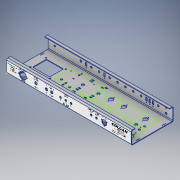
# Autodesk Inventor part: mainChassis
Saved by Autodesk Inventor 2018.3 (Build 223284000, 284)
## iProperties
Created: 2019-02-19
Part Number: mainChassis
Material: Aluminum 6061
Document SubType Name: Sheet Metal
Designer: RCCol
Density: 2.7 g/cm^3
Sheet Metal Rule: .125 thick aluminum
Appearance: Aluminum - Flat
Flat Pattern Width: 34.7497 cm
Flat Pattern Length: 60.325 cm
Flat Pattern Area: 2096.27 cm^2
Sheet Metal Width: 13.681 in
Sheet Metal Length: 23.750 in
Sheet Metal Area: 324.923 in^2
Author: RCCol
Autodesk Inventor part; units mm, degrees
(part 1 of 3)
ref_plane "YZ Plane" through (0, 0, 0) normal (1, 0, 0) x (0, 1, 0)
ref_plane "XZ Plane" through (0, 0, 0) normal (0, 1, 0) x (-1, 0, 0)
ref_plane "XY Plane" through (0, 0, 0) normal (0, 0, 1) x (1, 0, 0)
sketch "Sketch1" plane through (0, 0, 0) normal (0, 1, 0) x (-1, 0, 0)
  line L0 (0, 0) -> (-603.25, 0)
  line L1 (-603.25, 0) -> (-603.25, -204.47)
  line L2 (-603.25, -204.47) -> (0, -204.47)
  line L3 (0, -204.47) -> (0, 0)
  line L4 (0, 0) -> (-254, 0)
  line L5 (0, -79.375) -> (0, 0)
  dimension "d0" = 603.25
  dimension "d1" = 204.47
  constraints: 12 end point, 2 horizontal, 2 parallel, 1 perpendicular
  measures "d0" distance of L2.end L1.end
  measures "d1" distance of L1.end L0.end
extrude "Plate1" add sketch "Sketch1" along normal blind 3.175
sketch "Sketch2" plane through (0, 3.175, 0) normal (0, 1, 0) x (1, 0, 0)
  line L0 (41.3, 154.94) -> (117.45, 154.94)
  arc A0 (120.65, 151.74) -> (117.45, 154.94) centre (117.45, 151.74) ccw
  line L1 (41.3, 87.63) -> (117.45, 87.63)
  arc A1 (117.45, 87.63) -> (120.65, 90.83) centre (117.45, 90.83) ccw
  line L2 (38.1, 151.74) -> (38.1, 90.83)
  arc A2 (41.3, 154.94) -> (38.1, 151.74) centre (41.3, 151.74) ccw
  arc A3 (38.1, 90.83) -> (41.3, 87.63) centre (41.3, 90.83) ccw
  circle A4 centre (31.75, 177.5295) radius 1.5
  line L3 (120.65, 151.74) -> (120.65, 90.83)
  circle A5 centre (147.375, 75.2475) radius 1.65
  circle A6 centre (147.375, 164.1475) radius 1.65
  circle A7 centre (185.1575, 138.7475) radius 2.65
  circle A8 centre (185.1575, 178.435) radius 2.65
  circle A9 centre (235.9575, 87.1648) radius 2.65
  circle A10 centre (243.895, 87.1648) radius 2.65
  circle A11 centre (235.9575, 169.7148) radius 2.65
  circle A12 centre (243.895, 169.7148) radius 2.65
  circle A13 centre (259.135, 75.2475) radius 1.65
  circle A14 centre (259.135, 164.1475) radius 1.65
  circle A15 centre (551.549, 97.0569) radius 1.65
  arc A16 (187.6575, 169.4256) -> (182.6575, 169.4256) centre (185.1575, 169.4256) ccw
  arc A17 (182.6575, 164.4256) -> (187.6575, 164.4256) centre (185.1575, 164.4256) ccw
  line L4 (187.6575, 169.4256) -> (187.6575, 164.4256)
  line L5 (182.6575, 169.4256) -> (182.6575, 164.4256)
  arc A18 (187.6575, 90.4475) -> (182.6575, 90.4475) centre (185.1575, 90.4475) ccw
  arc A19 (182.6575, 85.4475) -> (187.6575, 85.4475) centre (185.1575, 85.4475) ccw
  line L6 (187.6575, 90.4475) -> (187.6575, 85.4475)
  line L7 (182.6575, 90.4475) -> (182.6575, 85.4475)
  arc A20 (308.1355, 175.935) -> (308.1355, 180.935) centre (308.1355, 178.435) ccw
  arc A21 (301.1355, 180.935) -> (301.1355, 175.935) centre (301.1355, 178.435) ccw
  line L8 (308.1355, 175.935) -> (301.1355, 175.935)
  line L9 (308.1355, 180.935) -> (301.1355, 180.935)
  arc A22 (243.048, 175.935) -> (243.048, 180.935) centre (243.048, 178.435) ccw
  arc A23 (236.048, 180.935) -> (236.048, 175.935) centre (236.048, 178.435) ccw
  line L10 (243.048, 175.935) -> (236.048, 175.935)
  line L11 (243.048, 180.935) -> (236.048, 180.935)
  arc A24 (298.195, 167.2148) -> (298.195, 172.2148) centre (298.195, 169.7148) ccw
  arc A25 (291.195, 172.2148) -> (291.195, 167.2148) centre (291.195, 169.7148) ccw
  line L12 (298.195, 167.2148) -> (291.195, 167.2148)
  line L13 (298.195, 172.2148) -> (291.195, 172.2148)
  arc A26 (308.1355, 110.435) -> (308.1355, 115.435) centre (308.1355, 112.935) ccw
  arc A27 (301.1355, 115.435) -> (301.1355, 110.435) centre (301.1355, 112.935) ccw
  line L14 (308.1355, 110.435) -> (301.1355, 110.435)
  line L15 (308.1355, 115.435) -> (301.1355, 115.435)
  arc A28 (308.1355, 99.735) -> (308.1355, 104.735) centre (308.1355, 102.235) ccw
  arc A29 (301.1355, 104.735) -> (301.1355, 99.735) centre (301.1355, 102.235) ccw
  line L16 (308.1355, 99.735) -> (301.1355, 99.735)
  line L17 (308.1355, 104.735) -> (301.1355, 104.735)
  arc A30 (243.048, 110.435) -> (243.048, 115.435) centre (243.048, 112.935) ccw
  arc A31 (236.048, 115.435) -> (236.048, 110.435) centre (236.048, 112.935) ccw
  line L18 (243.048, 110.435) -> (236.048, 110.435)
  line L19 (243.048, 115.435) -> (236.048, 115.435)
  arc A32 (243.048, 99.735) -> (243.048, 104.735) centre (243.048, 102.235) ccw
  arc A33 (236.048, 104.735) -> (236.048, 99.735) centre (236.048, 102.235) ccw
  line L20 (243.048, 99.735) -> (236.048, 99.735)
  line L21 (243.048, 104.735) -> (236.048, 104.735)
  arc A34 (298.195, 84.6648) -> (298.195, 89.6648) centre (298.195, 87.1648) ccw
  arc A35 (291.195, 89.6648) -> (291.195, 84.6648) centre (291.195, 87.1648) ccw
  line L22 (298.195, 84.6648) -> (291.195, 84.6648)
  line L23 (298.195, 89.6648) -> (291.195, 89.6648)
  circle A36 centre (237.6, 35.56) radius 15.1
  arc A37 (239.251, 57.4158) -> (238.6557, 58.0111) centre (238.6557, 57.4158) ccw
  arc A38 (238.6557, 53.1089) -> (239.251, 53.7042) centre (238.6557, 53.7042) ccw
  line L24 (239.251, 53.7042) -> (239.251, 57.4158)
  arc A39 (236.5443, 58.0111) -> (235.949, 57.4158) centre (236.5443, 57.4158) ccw
  line L25 (235.949, 53.7042) -> (235.949, 57.4158)
  line L26 (238.6557, 58.0111) -> (236.5443, 58.0111)
  line L27 (238.6557, 53.1089) -> (236.5443, 53.1089)
  arc A40 (235.949, 53.7042) -> (236.5443, 53.1089) centre (236.5443, 53.7042) ccw
  arc A41 (239.251, 17.4158) -> (238.6557, 18.0111) centre (238.6557, 17.4158) ccw
  arc A42 (238.6557, 13.1089) -> (239.251, 13.7042) centre (238.6557, 13.7042) ccw
  line L28 (239.251, 13.7042) -> (239.251, 17.4158)
  arc A43 (236.5443, 18.0111) -> (235.949, 17.4158) centre (236.5443, 17.4158) ccw
  line L29 (235.949, 13.7042) -> (235.949, 17.4158)
  line L30 (238.6557, 18.0111) -> (236.5443, 18.0111)
  line L31 (238.6557, 13.1089) -> (236.5443, 13.1089)
  arc A44 (235.949, 13.7042) -> (236.5443, 13.1089) centre (236.5443, 13.7042) ccw
  circle A45 centre (174.1, 35.56) radius 15.1
  arc A46 (175.751, 57.4158) -> (175.1557, 58.0111) centre (175.1557, 57.4158) ccw
  arc A47 (175.1557, 53.1089) -> (175.751, 53.7042) centre (175.1557, 53.7042) ccw
  line L32 (175.751, 53.7042) -> (175.751, 57.4158)
  arc A48 (173.0443, 58.0111) -> (172.449, 57.4158) centre (173.0443, 57.4158) ccw
  line L33 (172.449, 53.7042) -> (172.449, 57.4158)
  line L34 (175.1557, 58.0111) -> (173.0443, 58.0111)
  line L35 (175.1557, 53.1089) -> (173.0443, 53.1089)
  arc A49 (172.449, 53.7042) -> (173.0443, 53.1089) centre (173.0443, 53.7042) ccw
  arc A50 (175.751, 17.4158) -> (175.1557, 18.0111) centre (175.1557, 17.4158) ccw
  arc A51 (175.1557, 13.1089) -> (175.751, 13.7042) centre (175.1557, 13.7042) ccw
  line L36 (175.751, 13.7042) -> (175.751, 17.4158)
  arc A52 (173.0443, 18.0111) -> (172.449, 17.4158) centre (173.0443, 17.4158) ccw
  line L37 (172.449, 13.7042) -> (172.449, 17.4158)
  line L38 (175.1557, 18.0111) -> (173.0443, 18.0111)
  line L39 (175.1557, 13.1089) -> (173.0443, 13.1089)
  arc A53 (172.449, 13.7042) -> (173.0443, 13.1089) centre (173.0443, 13.7042) ccw
  circle A54 centre (110.6, 35.56) radius 15.1
  arc A55 (112.251, 57.4158) -> (111.6557, 58.0111) centre (111.6557, 57.4158) ccw
  arc A56 (111.6557, 53.1089) -> (112.251, 53.7042) centre (111.6557, 53.7042) ccw
  line L40 (112.251, 53.7042) -> (112.251, 57.4158)
  arc A57 (109.5443, 58.0111) -> (108.949, 57.4158) centre (109.5443, 57.4158) ccw
  line L41 (108.949, 53.7042) -> (108.949, 57.4158)
  line L42 (111.6557, 58.0111) -> (109.5443, 58.0111)
  line L43 (111.6557, 53.1089) -> (109.5443, 53.1089)
  arc A58 (108.949, 53.7042) -> (109.5443, 53.1089) centre (109.5443, 53.7042) ccw
  arc A59 (112.251, 17.4158) -> (111.6557, 18.0111) centre (111.6557, 17.4158) ccw
  arc A60 (111.6557, 13.1089) -> (112.251, 13.7042) centre (111.6557, 13.7042) ccw
  line L44 (112.251, 13.7042) -> (112.251, 17.4158)
  arc A61 (109.5443, 18.0111) -> (108.949, 17.4158) centre (109.5443, 17.4158) ccw
  line L45 (108.949, 13.7042) -> (108.949, 17.4158)
  line L46 (111.6557, 18.0111) -> (109.5443, 18.0111)
  line L47 (111.6557, 13.1089) -> (109.5443, 13.1089)
  arc A62 (108.949, 13.7042) -> (109.5443, 13.1089) centre (109.5443, 13.7042) ccw
  circle A63 centre (47.1, 35.56) radius 15.1
  arc A64 (48.751, 57.4158) -> (48.1557, 58.0111) centre (48.1557, 57.4158) ccw
  arc A65 (48.1557, 53.1089) -> (48.751, 53.7042) centre (48.1557, 53.7042) ccw
  line L48 (48.751, 53.7042) -> (48.751, 57.4158)
  arc A66 (46.0443, 58.0111) -> (45.449, 57.4158) centre (46.0443, 57.4158) ccw
  line L49 (45.449, 53.7042) -> (45.449, 57.4158)
  line L50 (48.1557, 58.0111) -> (46.0443, 58.0111)
  line L51 (48.1557, 53.1089) -> (46.0443, 53.1089)
  arc A67 (45.449, 53.7042) -> (46.0443, 53.1089) centre (46.0443, 53.7042) ccw
  arc A68 (48.751, 17.4158) -> (48.1557, 18.0111) centre (48.1557, 17.4158) ccw
  arc A69 (48.1557, 13.1089) -> (48.751, 13.7042) centre (48.1557, 13.7042) ccw
  line L52 (48.751, 13.7042) -> (48.751, 17.4158)
  arc A70 (46.0443, 18.0111) -> (45.449, 17.4158) centre (46.0443, 17.4158) ccw
  line L53 (45.449, 13.7042) -> (45.449, 17.4158)
  line L54 (48.1557, 18.0111) -> (46.0443, 18.0111)
  line L55 (48.1557, 13.1089) -> (46.0443, 13.1089)
  arc A71 (45.449, 13.7042) -> (46.0443, 13.1089) centre (46.0443, 13.7042) ccw
  circle A72 centre (159.7575, 106.3403) radius 4.8
  circle A73 centre (212.2, 93.5148) radius 4.8
  circle A74 centre (309.5568, 135.335) radius 6.35
  circle A75 centre (234.6268, 135.335) radius 6.35
  circle A76 centre (269.35, 26.9408) radius 1.651
  circle A77 centre (515.9375, 36.5125) radius 9.525
  circle A78 centre (515.3168, 50.7865) radius 1.651
  circle A79 centre (516.5582, 22.2385) radius 1.651
  circle A80 centre (530.225, 142.875) radius 9.525
  circle A81 centre (530.225, 157.1625) radius 1.651
  circle A82 centre (530.225, 128.5875) radius 1.651
  circle A83 centre (425.45, 142.875) radius 9.525
  circle A84 centre (425.45, 157.1625) radius 1.651
  circle A85 centre (425.45, 128.5875) radius 1.651
  circle A86 centre (363.5375, 142.875) radius 9.525
  circle A87 centre (363.5375, 157.1625) radius 1.651
  circle A88 centre (363.5375, 128.5875) radius 1.651
  circle A89 centre (336.55, 37.1475) radius 9.525
  circle A90 centre (336.757, 22.8615) radius 1.651
  circle A91 centre (336.343, 51.4335) radius 1.651
  circle A92 centre (205.85, 26.9408) radius 1.651
  circle A93 centre (78.85, 26.9408) radius 1.651
  circle A94 centre (78.85, 63.0879) radius 1.651
  circle A95 centre (19.05, 63.0879) radius 1.651
  circle A96 centre (142.35, 26.035) radius 1.651
  circle A97 centre (22.225, 20.5908) radius 1.651
  arc A98 (187.6575, 104.4569) -> (182.6575, 104.4569) centre (185.1575, 104.4569) ccw
  arc A99 (182.6575, 99.4569) -> (187.6575, 99.4569) centre (185.1575, 99.4569) ccw
  line L56 (187.6575, 104.4569) -> (187.6575, 99.4569)
  line L57 (182.6575, 104.4569) -> (182.6575, 99.4569)
  circle A100 centre (193.85, 60.5908) radius 1.65
  circle A101 centre (217.85, 60.5908) radius 1.65
  circle A102 centre (205.85, 60.5908) radius 4.826
  circle A103 centre (137.16, 62.3578) radius 1.651
  circle A104 centre (558.8, 109.5375) radius 4.826
  circle A105 centre (558.8, 84.1375) radius 4.826
  circle A106 centre (518.6157, 61.2782) radius 2.3813
  circle A107 centre (529.5939, 97.3765) radius 6.35
  circle A108 centre (563.0654, 61.4489) radius 2.3813
  circle A109 centre (31.75, 159.385) radius 3.175
  circle A110 centre (127, 159.385) radius 3.175
  circle A111 centre (31.75, 83.185) radius 3.175
  circle A112 centre (127, 83.185) radius 3.175
  circle A113 centre (565.8874, 37.1475) radius 9.525
  circle A114 centre (565.8026, 51.4347) radius 1.651
  circle A115 centre (565.9721, 22.8603) radius 1.651
  circle A116 centre (78.85, 35.56) radius 3.2385
  circle A117 centre (142.35, 35.56) radius 3.2385
  circle A118 centre (205.85, 35.56) radius 3.2385
  circle A119 centre (269.35, 35.56) radius 3.2385
  circle A120 centre (6.35, 165.735) radius 2.667
  circle A121 centre (6.35, 158.3944) radius 1.5875
  circle A122 centre (6.35, 173.0756) radius 1.5875
  circle A123 centre (6.35, 38.735) radius 2.667
  circle A124 centre (6.35, 31.3944) radius 1.5875
  circle A125 centre (6.35, 46.0756) radius 1.5875
  circle A126 centre (596.9, 38.735) radius 2.667
  circle A127 centre (596.9, 46.0756) radius 1.5875
  circle A128 centre (596.9, 31.3944) radius 1.5875
  circle A129 centre (596.9, 165.735) radius 2.667
  circle A130 centre (596.9, 173.0756) radius 1.5875
  circle A131 centre (596.9, 158.3944) radius 1.5875
  circle A132 centre (257.175, 61.9125) radius 3.2385
  circle A133 centre (117.45, 90.83) radius 3.2
  circle A134 centre (41.3, 90.83) radius 3.2
  circle A135 centre (41.3, 151.74) radius 3.2
  circle A136 centre (117.45, 151.74) radius 3.2
  line L58 (117.45, 87.63) -> (41.3, 87.63)
  line L59 (41.3, 87.63) -> (41.3, 154.94)
  line L60 (41.3, 154.94) -> (117.45, 154.94)
  line L61 (117.45, 154.94) -> (117.45, 87.63)
  line L62 (38.1, 90.83) -> (120.65, 90.83)
  line L63 (120.65, 90.83) -> (120.65, 151.74)
  line L64 (120.65, 151.74) -> (38.1, 151.74)
  line L65 (38.1, 151.74) -> (38.1, 90.83)
  line L66 (481.5672, 92.8982) -> (586.4692, 92.8982) construction
  line L67 (586.4692, 92.8982) -> (586.4692, 13.4373) construction
  line L68 (586.4692, 13.4373) -> (481.5672, 13.4373) construction
  line L69 (481.5672, 13.4373) -> (481.5672, 92.8982) construction
  line L70 (327.7837, 182.0084) -> (581.4999, 182.0084) construction
  line L71 (581.4999, 182.0084) -> (581.4999, 102.7644) construction
  line L72 (581.4999, 102.7644) -> (327.7837, 102.7644) construction
  line L73 (327.7837, 102.7644) -> (327.7837, 182.0084) construction
  line L74 (264.3245, 93.0716) -> (416.75, 93.5014) construction
  line L75 (416.75, 93.5014) -> (416.9742, 13.9788) construction
  line L76 (416.9742, 13.9788) -> (264.5487, 13.549) construction
  line L77 (264.5487, 13.549) -> (264.3245, 93.0716) construction
  circle A137 centre (298.195, 37.1475) radius 9.525
  circle A138 centre (298.3621, 51.434) radius 1.651
  circle A139 centre (298.0279, 22.861) radius 1.651
  line L78 (137.2091, 179.1073) -> (295.4903, 179.1073) construction
  line L79 (295.4903, 179.1073) -> (295.4903, 100.0089) construction
  line L80 (295.4903, 100.0089) -> (137.2091, 100.0089) construction
  line L81 (137.2091, 100.0089) -> (137.2091, 179.1073) construction
  circle A140 centre (436.5625, 46.0375) radius 14.9987
  circle A141 centre (436.5625, 68.8975) radius 1.651
  circle A142 centre (436.5625, 23.1775) radius 1.651
  dimension "GapSize" = 3.175
  dimension "d353" = 29.9974
  dimension "d378" = 3.302
  dimension "d379" = 3.302
  dimension "d417" = 22.86
  dimension "d418" = 22.86
  constraints: 141 centre point, 132 end point, 116 point on circle, 4 coincident, 4 parallel, 2 horizontal, 2 horizontal alignment, 2 perpendicular, 2 point on line, 12 other
  measures "d353" diameter of A140
  measures "d378" diameter of A141
  measures "d379" diameter of A142
  measures "d417" distance of A141.centre A140.centre
  measures "d418" distance of A140.centre A142.centre
extrude "Cut1" cut sketch "Sketch2" against normal blind 3.175 contours L59 L64 A2 | L0 A136 L64 A135 | A135 L64 L59 | L61 L64 A136 | A0 L64 L61 | A135 L59 A134 L2 | L64 L59 A135 | L64 A136 L61 A133 L62 A134 L59 A135 | A135 L59 L64 | L3 A133 L61 A136 | A136 L61 L64 | L64 L61 A136 | L62 L59 A3 | A134 L59 L62 | L62 L61 A133 | A1 L61 L62 | A134 L62 A133 L1 | L59 L62 A134 | A134 L62 L59 | A133 L62 L61 | L61 L62 A133 | A5 | A6 | A7 | A8 | A9 | A10 | A11 | A12 | A13 | A14 | A15 | L4 A17 L5 A16 | L6 A19 L7 A18 | L8 A21 L9 A20 | L10 A23 L11 A22 | L12 A25 L13 A24 | L14 A27 L15 A26 | L16 A29 L17 A28 | L18 A31 L19 A30 | L20 A33 L21 A32 | L22 A35 L23 A34 | A36 | L24 A38 L27 A40 L25 A39 L26 A37 | L28 A42 L31 A44 L29 A43 L30 A41 | A45 | L32 A47 L35 A49 L33 A48 L34 A46 | L36 A51 L39 A53 L37 A52 L38 A50 | A54 | L40 A56 L43 A58 L41 A57 L42 A55 | L44 A60 L47 A62 L45 A61 L46 A59 | A63 | L48 A65 L51 A67 L49 A66 L50 A64 | L52 A69 L55 A71 L53 A70 L54 A68 | A72 | A73 | A74 | A75 | A76 | A77 | A78 | A79 | A80 | A81 | A82 | A83 | A84 | A85 | A86 | A87 | A88 | A89 | A90 | A91 | A92 | A93 | A94 | A95 | A96 | A97 | L56 A99 L57 A98 | A100 | A101 | A102 | A103 | A104 | A105 | A106 | A107 | A108 | A109 | A110 | A111 | A112 | A113 | A114 | A115 | A116 | A117 | A118 | A119 | A120 | A121 | A122 | A123 | A124 | A125 | A126 | A127 | A128 | A129 | A130 | A131 | A132 | A137 | A138 | A139 | A140 | A141 | A142
sketch "Sketch3" plane through (603.25, 0, -3.175) normal (0, 0, 1) x (1, 0, 0)
  line L0 (-603.25, 0) -> (0, 0)
  line L1 (0, 0) -> (0, 63.5)
  line L2 (0, 63.5) -> (-603.25, 63.5)
  line L3 (-603.25, 63.5) -> (-603.25, 0)
  constraints: 6 end point, 1 horizontal, 1 perpendicular, 1 vertical
edge flange "Flange1" height 63.5 angle 90 thickness 3.175 bend radius 3.175 thickness toward (0, 0, 1) relief straight relief width 3.175 relief depth 1.5875 edges at (301.625, 3.175, 0) wall of the first edge with corners at (0, 0, -3.175) (603.25, 0, -3.175) (603.25, 63.5, -3.175) (0, 63.5, -3.175)
bend "Bend1"
corner "Corner1"
sketch "Sketch4" plane through (603.25, 60.325, 0) normal (0, 1, 0) x (-1, 0, 0)
  line L0 (603.25, 0) -> (0, 0)
  line L1 (0, 0) -> (0, -19.05)
  line L2 (0, -19.05) -> (603.25, -19.05)
  line L3 (603.25, -19.05) -> (603.25, 0)
  constraints: 6 end point, 1 horizontal, 1 perpendicular, 1 vertical
edge flange "Flange2" height 19.05 angle 90 thickness 3.175 bend radius 3.175 thickness toward (0, 1, 0) relief straight relief width 3.175 relief depth 1.5875 edges at (301.625, 63.5, -3.175) wall of the first edge with corners at (0, 60.325, 0) (603.25, 60.325, 0) (603.25, 60.325, -19.05) (0, 60.325, -19.05)
bend "Bend2"
corner "Corner2"
sketch "Sketch5" plane through (0, 6.35, 0) normal (0, 0, 1) x (1, 0, 0)
  circle A0 centre (78.85, 25.4) radius 17.4625
  circle A1 centre (99.805, 25.4) radius 1.778
  circle A2 centre (57.895, 25.4) radius 1.778
  line L0 (148.065, 22.0907) -> (148.065, 28.7093)
  line L1 (136.635, 22.0907) -> (136.635, 28.7093)
  arc A3 (136.635, 22.0907) -> (148.065, 22.0907) centre (142.35, 25.4) ccw
  arc A4 (148.065, 28.7093) -> (136.635, 28.7093) centre (142.35, 25.4) ccw
  line L2 (193.9018, 20.2386) -> (192.3982, 20.2386)
  arc A5 (193.9018, 19.2226) -> (192.3982, 19.2226) centre (193.15, 25.4) ccw
  line L3 (192.3982, 20.2386) -> (192.3982, 19.2226)
  line L4 (193.9018, 19.2226) -> (193.9018, 20.2386)
  line L5 (219.3018, 20.2386) -> (217.7982, 20.2386)
  arc A6 (219.3018, 19.2226) -> (217.7982, 19.2226) centre (218.55, 25.4) ccw
  line L6 (217.7982, 20.2386) -> (217.7982, 19.2226)
  line L7 (219.3018, 19.2226) -> (219.3018, 20.2386)
  circle A7 centre (261.3213, 25.4) radius 4.7625
  circle A8 centre (286.7213, 25.4) radius 4.7625
  circle A9 centre (312.1213, 25.4) radius 4.7625
  circle A10 centre (409.575, 25.5399) radius 4.7625
  circle A11 centre (434.975, 25.5399) radius 4.7625
  circle A12 centre (473.075, 25.5399) radius 12.1031
  circle A13 centre (460.2734, 32.9821) radius 1.778
  circle A14 centre (485.8766, 32.9821) radius 1.778
  circle A15 centre (473.075, 10.7317) radius 1.778
  line L8 (136.635, 28.7093) -> (148.065, 28.7093)
  line L9 (148.065, 28.7093) -> (148.065, 22.0907)
  line L10 (148.065, 22.0907) -> (136.635, 22.0907)
  line L11 (136.635, 22.0907) -> (136.635, 28.7093)
  arc A16 (148.065, 28.7093) -> (136.635, 28.7093) centre (142.35, 25.4) ccw
  arc A17 (136.635, 22.0907) -> (148.065, 22.0907) centre (142.35, 25.4) ccw
  arc A18 (136.635, 22.0907) -> (148.065, 22.0907) centre (142.35, 25.4) ccw
  arc A19 (193.9018, 19.2226) -> (192.3982, 19.2226) centre (193.15, 25.4) ccw
  line L12 (193.9018, 19.2226) -> (193.9018, 20.2386)
  line L13 (192.3982, 20.2386) -> (192.3982, 19.2226)
  point P0 (0, -6.35)
  dimension "GapSize" = 3.175
  constraints: 28 end point, 23 point on circle, 20 centre point, 5 point on line, 2 parallel, 1 concentric, 1 horizontal, 1 perpendicular, 1 vertical
extrude "Cut2" cut sketch "Sketch5" against normal blind 3.175
sketch "Sketch6" plane through (0, 0, -201.295) normal (0, 0, -1) x (-1, 0, 0)
  line L0 (-603.25, 0) -> (0, 0)
  line L1 (0, 0) -> (0, 63.5)
  line L2 (0, 63.5) -> (-603.25, 63.5)
  line L3 (-603.25, 63.5) -> (-603.25, 0)
  constraints: 6 end point, 1 horizontal, 1 perpendicular, 1 vertical
edge flange "Flange3" height 63.5 angle 90 thickness 3.175 bend radius 3.175 thickness toward (0, 0, -1) relief straight relief width 3.175 relief depth 1.5875 edges at (301.625, 3.175, -204.47) wall of the first edge with corners at (603.25, 0, -201.295) (0, 0, -201.295) (0, 63.5, -201.295) (603.25, 63.5, -201.295)
bend "Bend3"
corner "Corner3"
sketch "Sketch7" plane through (0, 60.325, -204.47) normal (0, 1, 0) x (-1, 0, 0)
  line L0 (-603.25, 0) -> (0, 0)
  line L1 (0, 0) -> (0, 19.05)
  line L2 (0, 19.05) -> (-603.25, 19.05)
  line L3 (-603.25, 19.05) -> (-603.25, 0)
  constraints: 6 end point, 1 horizontal, 1 perpendicular, 1 vertical
edge flange "Flange4" height 19.05 angle 90 thickness 3.175 bend radius 3.175 thickness toward (0, 1, 0) relief straight relief width 3.175 relief depth 1.5875 edges at (301.625, 63.5, -201.295) wall of the first edge with corners at (603.25, 60.325, -204.47) (0, 60.325, -204.47) (0, 60.325, -185.42) (603.25, 60.325, -185.42)
bend "Bend4"
corner "Corner4"
sketch "Sketch8" plane through (603.25, 6.35, -204.47) normal (0, 0, -1) x (-1, 0, 0)
  line L0 (0, -6.35) -> (603.25, -6.35)
  line L1 (603.25, -6.35) -> (603.25, 57.15)
  line L2 (603.25, 57.15) -> (0, 57.15)
  line L3 (0, 57.15) -> (0, -6.35)
  circle A0 centre (31.9541, 38.1) radius 4.7625
  circle A1 centre (70.0541, 25.4) radius 4.7625
  circle A2 centre (190.9581, 25.4) radius 4.7625
  circle A3 centre (305.2581, 25.4) radius 4.7625
  circle A4 centre (444.9581, 25.4) radius 4.7625
  circle A5 centre (394.1581, 25.4) radius 4.7625
  circle A6 centre (356.0581, 25.4) radius 4.7625
  circle A7 centre (267.1581, 25.4) radius 4.7625
  circle A8 centre (229.0581, 25.4) radius 4.7625
  circle A9 centre (152.8581, 25.4) radius 4.7625
  circle A10 centre (31.9541, 12.7) radius 4.7625
  circle A11 centre (31.9541, 12.7) radius 4.7625
  circle A12 centre (152.8581, 25.4) radius 4.7625
  circle A13 centre (229.0581, 25.4) radius 4.7625
  circle A14 centre (267.1581, 25.4) radius 4.7625
  circle A15 centre (356.0581, 25.4) radius 4.7625
  circle A16 centre (394.1581, 25.4) radius 4.7625
  circle A17 centre (444.9581, 25.4) radius 4.7625
  circle A18 centre (305.2581, 25.4) radius 4.7625
  circle A19 centre (190.9581, 25.4) radius 4.7625
  circle A20 centre (70.0541, 25.4) radius 4.7625
  circle A21 centre (31.9541, 38.1) radius 4.7625
  circle A22 centre (571.5, 25.4) radius 3.9624
  circle A23 centre (95.4541, 39.6875) radius 1.7272
  circle A24 centre (95.4541, 11.1125) radius 1.7272
  line L4 (91.4854, 18.2562) -> (91.4854, 32.5437)
  line L5 (91.4854, 32.5437) -> (99.4229, 32.5438)
  line L6 (99.4229, 32.5438) -> (99.4229, 18.2563)
  line L7 (99.4229, 18.2563) -> (91.4854, 18.2562)
  circle A25 centre (111.4561, 39.6875) radius 1.7272
  circle A26 centre (111.4561, 11.1125) radius 1.7272
  line L8 (107.4874, 18.2562) -> (107.4874, 32.5437)
  line L9 (107.4874, 32.5437) -> (115.4249, 32.5438)
  line L10 (115.4249, 32.5438) -> (115.4249, 18.2563)
  line L11 (115.4249, 18.2563) -> (107.4874, 18.2562)
  circle A27 centre (127.4581, 39.6875) radius 1.7272
  circle A28 centre (127.4581, 11.1125) radius 1.7272
  line L12 (123.4894, 18.2562) -> (123.4894, 32.5437)
  line L13 (123.4894, 32.5437) -> (131.4269, 32.5438)
  line L14 (131.4269, 32.5438) -> (131.4269, 18.2563)
  line L15 (131.4269, 18.2563) -> (123.4894, 18.2562)
  circle A29 centre (330.6581, 39.6875) radius 1.7272
  circle A30 centre (330.6581, 11.1125) radius 1.7272
  line L16 (326.6894, 18.2562) -> (326.6894, 32.5437)
  line L17 (326.6894, 32.5437) -> (334.6269, 32.5438)
  line L18 (334.6269, 32.5438) -> (334.6269, 18.2563)
  line L19 (334.6269, 18.2563) -> (326.6894, 18.2562)
  circle A31 centre (419.5581, 39.6875) radius 1.7272
  circle A32 centre (419.5581, 11.1125) radius 1.7272
  line L20 (415.5894, 18.2562) -> (415.5894, 32.5437)
  line L21 (415.5894, 32.5437) -> (423.5269, 32.5438)
  line L22 (423.5269, 32.5438) -> (423.5269, 18.2563)
  line L23 (423.5269, 18.2563) -> (415.5894, 18.2562)
  dimension "GapSize" = 3.175
  constraints: 48 end point, 33 centre point
extrude "Cut3" cut sketch "Sketch8" against normal blind 3.175 contours A0 | A1 | A2 | A3 | A4 | A5 | A6 | A7 | A8 | A9 | A10 | A22 | A23 | A24 | L4 L5 L6 L7 | A25 | A26 | L8 L9 L10 L11 | A27 | A28 | L12 L13 L14 L15 | A29 | A30 | L16 L17 L18 L19 | A31 | A32 | L20 L21 L22 L23
sketch "Sketch9" plane through (603.25, 6.35, -204.47) normal (0, 0, -1) x (-1, 0, 0)
  line L0 (0, 50.8) -> (0, 53.975) projected
  line L1 (0, 53.975) -> (603.25, 53.975) projected
  line L2 (603.25, 53.975) -> (0, 53.975) projected
  line L3 (0, 50.8) -> (0, 0) projected
  line L4 (0, 50.8) -> (0, 0) projected
  line L5 (0, 50.8) -> (603.2512, 50.8) construction
  line L6 (603.2512, 50.8) -> (603.2512, -0.0001) construction
  line L7 (603.2512, -0.0001) -> (0, -0.0001) construction
  line L8 (0, -0.0001) -> (0, 50.8) construction
  point P0 (603.25, -6.35)
  constraints: 2 other
decal "Decal1"
sketch "Sketch10" plane through (0, 6.35, 0) normal (0, 0, 1) x (1, 0, 0)
  line L0 (0, 53.975) -> (0, 50.8) projected
  line L1 (0, 53.975) -> (603.2512, 53.975) construction
  line L2 (603.2512, 53.975) -> (603.2512, -3.1751) construction
  line L3 (603.2512, -3.1751) -> (0, -3.1751) construction
  line L4 (0, -3.1751) -> (0, 53.975) construction
  point P0 (0, -6.35)
  constraints: 2 other
decal "Decal2"
sketch "Sketch11" plane through (0, 3.175, 0) normal (0, 1, 0) x (1, 0, 0)
  line L0 (327.7837, 182.0084) -> (581.4999, 182.0084) construction
  line L1 (581.4999, 182.0084) -> (581.4999, 102.7644) construction
  line L2 (581.4999, 102.7644) -> (327.7837, 102.7644) construction
  line L3 (327.7837, 102.7644) -> (327.7837, 182.0084) construction
  line L4 (137.2091, 179.1073) -> (295.4903, 179.1073) construction
  line L5 (295.4903, 179.1073) -> (295.4903, 100.0089) construction
  line L6 (295.4903, 100.0089) -> (137.2091, 100.0089) construction
  line L7 (137.2091, 100.0089) -> (137.2091, 179.1073) construction
  line L8 (481.5672, 92.8982) -> (586.4692, 92.8982) construction
  line L9 (586.4692, 92.8982) -> (586.4692, 13.4373) construction
  line L10 (586.4692, 13.4373) -> (481.5672, 13.4373) construction
  line L11 (481.5672, 13.4373) -> (481.5672, 92.8982) construction
  point P0 (0, 0)
  constraints: 6 other
sketch "Sketch12" plane through (0, 3.175, 0) normal (0, 1, 0) x (1, 0, 0)
  line L0 (474.6625, 93.6574) -> (579.4451, 93.6574)
  line L1 (579.4451, 93.6574) -> (579.4451, 14.2875)
  line L2 (579.4451, 14.2875) -> (474.6625, 14.2875)
  line L3 (474.6625, 14.2875) -> (474.6625, 93.6574)
  line L4 (499.8974, 36.9392) -> (499.9406, 37.8409)
  line L5 (499.9406, 37.8409) -> (500.0676, 38.7375)
  line L6 (500.0676, 38.7375) -> (500.2809, 39.6189)
  line L7 (500.2809, 39.6189) -> (500.5781, 40.4749)
  line L8 (500.5781, 40.4749) -> (500.9566, 41.3004)
  line L9 (500.9566, 41.3004) -> (501.4087, 42.0827)
  line L10 (501.4087, 42.0827) -> (501.9319, 42.8193)
  line L11 (501.9319, 42.8193) -> (502.5263, 43.5051)
  line L12 (502.5263, 43.5051) -> (503.1816, 44.1274)
  line L13 (503.1816, 44.1274) -> (503.8903, 44.6888)
  line L14 (503.8903, 44.6888) -> (504.6523, 45.1764)
  line L15 (504.6523, 45.1764) -> (505.46, 45.593)
  line L16 (505.46, 45.593) -> (506.3007, 45.9283)
  line L17 (506.3007, 45.9283) -> (507.1669, 46.1848)
  line L18 (507.1669, 46.1848) -> (508.0559, 46.355)
  line L19 (508.0559, 46.355) -> (508.9576, 46.4439)
  line L20 (508.9576, 46.4439) -> (509.8669, 46.4439)
  line L21 (509.8669, 46.4439) -> (510.7686, 46.355)
  line L22 (510.7686, 46.355) -> (511.6551, 46.1848)
  line L23 (511.6551, 46.1848) -> (512.5237, 45.9283)
  line L24 (512.5237, 45.9283) -> (513.3619, 45.593)
  line L25 (513.3619, 45.593) -> (514.1671, 45.1764)
  line L26 (514.1671, 45.1764) -> (514.9291, 44.6888)
  line L27 (514.9291, 44.6888) -> (515.6429, 44.1274)
  line L28 (515.6429, 44.1274) -> (516.2982, 43.5051)
  line L29 (516.2982, 43.5051) -> (516.89, 42.8193)
  line L30 (516.89, 42.8193) -> (517.4158, 42.0827)
  line L31 (517.4158, 42.0827) -> (517.8679, 41.3004)
  line L32 (517.8679, 41.3004) -> (518.2489, 40.4749)
  line L33 (518.2489, 40.4749) -> (518.5385, 39.6189)
  line L34 (518.5385, 39.6189) -> (518.7544, 38.7375)
  line L35 (518.7544, 38.7375) -> (518.8839, 37.8409)
  line L36 (518.8839, 37.8409) -> (518.9271, 36.9392)
  line L37 (518.9271, 36.9392) -> (518.8839, 36.0324)
  line L38 (518.8839, 36.0324) -> (518.7544, 35.1358)
  line L39 (518.7544, 35.1358) -> (518.5385, 34.257)
  line L40 (518.5385, 34.257) -> (518.2489, 33.401)
  line L41 (518.2489, 33.401) -> (517.8679, 32.578)
  line L42 (517.8679, 32.578) -> (517.4158, 31.7957)
  line L43 (517.4158, 31.7957) -> (516.89, 31.0591)
  line L44 (516.89, 31.0591) -> (516.2982, 30.3733)
  line L45 (516.2982, 30.3733) -> (515.6429, 29.7459)
  line L46 (515.6429, 29.7459) -> (514.9291, 29.1897)
  line L47 (514.9291, 29.1897) -> (514.1671, 28.6969)
  line L48 (514.1671, 28.6969) -> (513.3619, 28.2829)
  line L49 (513.3619, 28.2829) -> (512.5237, 27.9476)
  line L50 (512.5237, 27.9476) -> (511.6551, 27.6936)
  line L51 (511.6551, 27.6936) -> (510.7686, 27.5209)
  line L52 (510.7686, 27.5209) -> (509.8669, 27.4345)
  line L53 (509.8669, 27.4345) -> (508.9576, 27.4345)
  line L54 (508.9576, 27.4345) -> (508.0559, 27.5209)
  line L55 (508.0559, 27.5209) -> (507.1669, 27.6936)
  line L56 (507.1669, 27.6936) -> (506.3007, 27.9476)
  line L57 (506.3007, 27.9476) -> (505.46, 28.2829)
  line L58 (505.46, 28.2829) -> (504.6523, 28.6969)
  line L59 (504.6523, 28.6969) -> (503.8903, 29.1897)
  line L60 (503.8903, 29.1897) -> (503.1816, 29.7459)
  line L61 (503.1816, 29.7459) -> (502.5263, 30.3733)
  line L62 (502.5263, 30.3733) -> (501.9319, 31.0591)
  line L63 (501.9319, 31.0591) -> (501.4087, 31.7957)
  line L64 (501.4087, 31.7957) -> (500.9566, 32.578)
  line L65 (500.9566, 32.578) -> (500.5781, 33.401)
  line L66 (500.5781, 33.401) -> (500.2809, 34.257)
  line L67 (500.2809, 34.257) -> (500.0676, 35.1358)
  line L68 (500.0676, 35.1358) -> (499.9406, 36.0324)
  line L69 (499.9406, 36.0324) -> (499.8974, 36.9392)
  line L70 (549.7906, 37.5742) -> (549.8338, 38.4759)
  line L71 (549.8338, 38.4759) -> (549.9633, 39.3725)
  line L72 (549.9633, 39.3725) -> (550.1767, 40.2514)
  line L73 (550.1767, 40.2514) -> (550.4713, 41.1099)
  line L74 (550.4713, 41.1099) -> (550.8498, 41.9303)
  line L75 (550.8498, 41.9303) -> (551.2994, 42.7177)
  line L76 (551.2994, 42.7177) -> (551.8252, 43.4543)
  line L77 (551.8252, 43.4543) -> (552.4195, 44.1401)
  line L78 (552.4195, 44.1401) -> (553.0748, 44.7624)
  line L79 (553.0748, 44.7624) -> (553.7886, 45.3212)
  line L80 (553.7886, 45.3212) -> (554.5506, 45.8114)
  line L81 (554.5506, 45.8114) -> (555.3532, 46.228)
  line L82 (555.3532, 46.228) -> (556.194, 46.5633)
  line L83 (556.194, 46.5633) -> (557.0626, 46.8198)
  line L84 (557.0626, 46.8198) -> (557.9516, 46.99)
  line L85 (557.9516, 46.99) -> (558.8533, 47.0738)
  line L86 (558.8533, 47.0738) -> (559.7576, 47.0738)
  line L87 (559.7576, 47.0738) -> (560.6593, 46.99)
  line L88 (560.6593, 46.99) -> (561.5483, 46.8198)
  line L89 (561.5483, 46.8198) -> (562.4195, 46.5633)
  line L90 (562.4195, 46.5633) -> (563.2552, 46.228)
  line L91 (563.2552, 46.228) -> (564.0629, 45.8114)
  line L92 (564.0629, 45.8114) -> (564.8223, 45.3212)
  line L93 (564.8223, 45.3212) -> (565.5361, 44.7624)
  line L94 (565.5361, 44.7624) -> (566.1914, 44.1401)
  line L95 (566.1914, 44.1401) -> (566.7832, 43.4543)
  line L96 (566.7832, 43.4543) -> (567.309, 42.7177)
  line L97 (567.309, 42.7177) -> (567.7611, 41.9303)
  line L98 (567.7611, 41.9303) -> (568.1396, 41.1099)
  line L99 (568.1396, 41.1099) -> (568.4342, 40.2514)
  line L100 (568.4342, 40.2514) -> (568.6476, 39.3725)
  line L101 (568.6476, 39.3725) -> (568.7771, 38.4759)
  line L102 (568.7771, 38.4759) -> (568.8203, 37.5742)
  line L103 (568.8203, 37.5742) -> (568.7771, 36.6674)
  line L104 (568.7771, 36.6674) -> (568.6476, 35.7708)
  line L105 (568.6476, 35.7708) -> (568.4342, 34.892)
  line L106 (568.4342, 34.892) -> (568.1396, 34.036)
  line L107 (568.1396, 34.036) -> (567.7611, 33.213)
  line L108 (567.7611, 33.213) -> (567.309, 32.4282)
  line L109 (567.309, 32.4282) -> (566.7832, 31.689)
  line L110 (566.7832, 31.689) -> (566.1914, 31.0058)
  line L111 (566.1914, 31.0058) -> (565.5361, 30.3809)
  line L112 (565.5361, 30.3809) -> (564.8223, 29.8221)
  line L113 (564.8223, 29.8221) -> (564.0629, 29.3319)
  line L114 (564.0629, 29.3319) -> (563.2552, 28.9179)
  line L115 (563.2552, 28.9179) -> (562.4195, 28.5826)
  line L116 (562.4195, 28.5826) -> (561.5483, 28.3286)
  line L117 (561.5483, 28.3286) -> (560.6593, 28.1559)
  line L118 (560.6593, 28.1559) -> (559.7576, 28.0695)
  line L119 (559.7576, 28.0695) -> (558.8533, 28.0695)
  line L120 (558.8533, 28.0695) -> (557.9516, 28.1559)
  line L121 (557.9516, 28.1559) -> (557.0626, 28.3286)
  line L122 (557.0626, 28.3286) -> (556.194, 28.5826)
  line L123 (556.194, 28.5826) -> (555.3532, 28.9179)
  line L124 (555.3532, 28.9179) -> (554.5506, 29.3319)
  line L125 (554.5506, 29.3319) -> (553.7886, 29.8221)
  line L126 (553.7886, 29.8221) -> (553.0748, 30.3809)
  line L127 (553.0748, 30.3809) -> (552.4195, 31.0058)
  line L128 (552.4195, 31.0058) -> (551.8252, 31.689)
  line L129 (551.8252, 31.689) -> (551.2994, 32.4282)
  line L130 (551.2994, 32.4282) -> (550.8498, 33.213)
  line L131 (550.8498, 33.213) -> (550.4713, 34.036)
  line L132 (550.4713, 34.036) -> (550.1767, 34.892)
  line L133 (550.1767, 34.892) -> (549.9633, 35.7708)
  line L134 (549.9633, 35.7708) -> (549.8338, 36.6674)
  line L135 (549.8338, 36.6674) -> (549.7906, 37.5742)
  line L136 (481.7948, 18.1204) -> (481.7903, 17.9914)
  line L137 (481.7903, 17.9914) -> (481.7768, 17.863)
  line L138 (481.7768, 17.863) -> (481.7544, 17.7359)
  line L139 (481.7544, 17.7359) -> (481.7232, 17.6107)
  line L140 (481.7232, 17.6107) -> (481.6833, 17.4879)
  line L141 (481.6833, 17.4879) -> (481.635, 17.3683)
  line L142 (481.635, 17.3683) -> (481.5784, 17.2523)
  line L143 (481.5784, 17.2523) -> (481.5138, 17.1405)
  line L144 (481.5138, 17.1405) -> (481.4417, 17.0335)
  line L145 (481.4417, 17.0335) -> (481.3622, 16.9318)
  line L146 (481.3622, 16.9318) -> (481.2758, 16.8359)
  line L147 (481.2758, 16.8359) -> (481.183, 16.7462)
  line L148 (481.183, 16.7462) -> (481.0841, 16.6632)
  line L149 (481.0841, 16.6632) -> (480.9797, 16.5874)
  line L150 (480.9797, 16.5874) -> (480.8703, 16.519)
  line L151 (480.8703, 16.519) -> (480.7563, 16.4584)
  line L152 (480.7563, 16.4584) -> (480.6384, 16.4059)
  line L153 (480.6384, 16.4059) -> (480.5171, 16.3617)
  line L154 (480.5171, 16.3617) -> (480.393, 16.3262)
  line L155 (480.393, 16.3262) -> (480.2668, 16.2993)
  line L156 (480.2668, 16.2993) -> (480.139, 16.2814)
  line L157 (480.139, 16.2814) -> (480.0102, 16.2724)
  line L158 (480.0102, 16.2724) -> (479.8812, 16.2724)
  line L159 (479.8812, 16.2724) -> (479.7524, 16.2814)
  line L160 (479.7524, 16.2814) -> (479.6246, 16.2993)
  line L161 (479.6246, 16.2993) -> (479.4984, 16.3262)
  line L162 (479.4984, 16.3262) -> (479.3743, 16.3617)
  line L163 (479.3743, 16.3617) -> (479.253, 16.4059)
  line L164 (479.253, 16.4059) -> (479.1351, 16.4584)
  line L165 (479.1351, 16.4584) -> (479.0211, 16.519)
  line L166 (479.0211, 16.519) -> (478.9117, 16.5874)
  line L167 (478.9117, 16.5874) -> (478.8073, 16.6632)
  line L168 (478.8073, 16.6632) -> (478.7084, 16.7462)
  line L169 (478.7084, 16.7462) -> (478.6156, 16.8359)
  line L170 (478.6156, 16.8359) -> (478.5292, 16.9318)
  line L171 (478.5292, 16.9318) -> (478.4497, 17.0335)
  line L172 (478.4497, 17.0335) -> (478.3776, 17.1405)
  line L173 (478.3776, 17.1405) -> (478.313, 17.2523)
  line L174 (478.313, 17.2523) -> (478.2564, 17.3683)
  line L175 (478.2564, 17.3683) -> (478.2081, 17.4879)
  line L176 (478.2081, 17.4879) -> (478.1682, 17.6107)
  line L177 (478.1682, 17.6107) -> (478.137, 17.7359)
  line L178 (478.137, 17.7359) -> (478.1146, 17.863)
  line L179 (478.1146, 17.863) -> (478.1011, 17.9914)
  line L180 (478.1011, 17.9914) -> (478.0966, 18.1204)
  line L181 (478.0966, 18.1204) -> (478.1011, 18.2493)
  line L182 (478.1011, 18.2493) -> (478.1146, 18.3777)
  line L183 (478.1146, 18.3777) -> (478.137, 18.5048)
  line L184 (478.137, 18.5048) -> (478.1682, 18.63)
  line L185 (478.1682, 18.63) -> (478.2081, 18.7528)
  line L186 (478.2081, 18.7528) -> (478.2564, 18.8725)
  line L187 (478.2564, 18.8725) -> (478.313, 18.9885)
  line L188 (478.313, 18.9885) -> (478.3776, 19.1002)
  line L189 (478.3776, 19.1002) -> (478.4497, 19.2072)
  line L190 (478.4497, 19.2072) -> (478.5292, 19.309)
  line L191 (478.5292, 19.309) -> (478.6156, 19.4049)
  line L192 (478.6156, 19.4049) -> (478.7084, 19.4945)
  line L193 (478.7084, 19.4945) -> (478.8073, 19.5775)
  line L194 (478.8073, 19.5775) -> (478.9117, 19.6533)
  line L195 (478.9117, 19.6533) -> (479.0211, 19.7217)
  line L196 (479.0211, 19.7217) -> (479.1351, 19.7823)
  line L197 (479.1351, 19.7823) -> (479.253, 19.8348)
  line L198 (479.253, 19.8348) -> (479.3743, 19.879)
  line L199 (479.3743, 19.879) -> (479.4984, 19.9146)
  line L200 (479.4984, 19.9146) -> (479.6246, 19.9414)
  line L201 (479.6246, 19.9414) -> (479.7524, 19.9594)
  line L202 (479.7524, 19.9594) -> (479.8812, 19.9684)
  line L203 (479.8812, 19.9684) -> (480.0102, 19.9684)
  line L204 (480.0102, 19.9684) -> (480.139, 19.9594)
  line L205 (480.139, 19.9594) -> (480.2668, 19.9414)
  line L206 (480.2668, 19.9414) -> (480.393, 19.9146)
  line L207 (480.393, 19.9146) -> (480.5171, 19.879)
  line L208 (480.5171, 19.879) -> (480.6384, 19.8348)
  line L209 (480.6384, 19.8348) -> (480.7563, 19.7823)
  line L210 (480.7563, 19.7823) -> (480.8703, 19.7217)
  line L211 (480.8703, 19.7217) -> (480.9797, 19.6533)
  line L212 (480.9797, 19.6533) -> (481.0841, 19.5775)
  line L213 (481.0841, 19.5775) -> (481.183, 19.4945)
  line L214 (481.183, 19.4945) -> (481.2758, 19.4049)
  line L215 (481.2758, 19.4049) -> (481.3622, 19.309)
  line L216 (481.3622, 19.309) -> (481.4417, 19.2072)
  line L217 (481.4417, 19.2072) -> (481.5138, 19.1002)
  line L218 (481.5138, 19.1002) -> (481.5784, 18.9885)
  line L219 (481.5784, 18.9885) -> (481.635, 18.8725)
  line L220 (481.635, 18.8725) -> (481.6833, 18.7528)
  line L221 (481.6833, 18.7528) -> (481.7232, 18.63)
  line L222 (481.7232, 18.63) -> (481.7544, 18.5048)
  line L223 (481.7544, 18.5048) -> (481.7768, 18.3777)
  line L224 (481.7768, 18.3777) -> (481.7903, 18.2493)
  line L225 (481.7903, 18.2493) -> (481.7948, 18.1204)
  line L226 (481.7974, 88.8746) -> (481.7929, 88.7456)
  line L227 (481.7929, 88.7456) -> (481.7794, 88.6173)
  line L228 (481.7794, 88.6173) -> (481.757, 88.4901)
  line L229 (481.757, 88.4901) -> (481.7257, 88.3649)
  line L230 (481.7257, 88.3649) -> (481.6858, 88.2422)
  line L231 (481.6858, 88.2422) -> (481.6375, 88.1225)
  line L232 (481.6375, 88.1225) -> (481.5809, 88.0065)
  line L233 (481.5809, 88.0065) -> (481.5164, 87.8947)
  line L234 (481.5164, 87.8947) -> (481.4442, 87.7877)
  line L235 (481.4442, 87.7877) -> (481.3647, 87.686)
  line L236 (481.3647, 87.686) -> (481.2784, 87.5901)
  line L237 (481.2784, 87.5901) -> (481.1855, 87.5004)
  line L238 (481.1855, 87.5004) -> (481.0867, 87.4175)
  line L239 (481.0867, 87.4175) -> (480.9823, 87.3416)
  line L240 (480.9823, 87.3416) -> (480.8728, 87.2732)
  line L241 (480.8728, 87.2732) -> (480.7588, 87.2126)
  line L242 (480.7588, 87.2126) -> (480.6409, 87.1601)
  line L243 (480.6409, 87.1601) -> (480.5196, 87.116)
  line L244 (480.5196, 87.116) -> (480.3956, 87.0804)
  line L245 (480.3956, 87.0804) -> (480.2693, 87.0536)
  line L246 (480.2693, 87.0536) -> (480.1415, 87.0356)
  line L247 (480.1415, 87.0356) -> (480.0128, 87.0266)
  line L248 (480.0128, 87.0266) -> (479.8837, 87.0266)
  line L249 (479.8837, 87.0266) -> (479.755, 87.0356)
  line L250 (479.755, 87.0356) -> (479.6271, 87.0536)
  line L251 (479.6271, 87.0536) -> (479.5009, 87.0804)
  line L252 (479.5009, 87.0804) -> (479.3768, 87.116)
  line L253 (479.3768, 87.116) -> (479.2555, 87.1601)
  line L254 (479.2555, 87.1601) -> (479.1376, 87.2126)
  line L255 (479.1376, 87.2126) -> (479.0237, 87.2732)
  line L256 (479.0237, 87.2732) -> (478.9142, 87.3416)
  line L257 (478.9142, 87.3416) -> (478.8098, 87.4175)
  line L258 (478.8098, 87.4175) -> (478.7109, 87.5004)
  line L259 (478.7109, 87.5004) -> (478.6181, 87.5901)
  line L260 (478.6181, 87.5901) -> (478.5317, 87.686)
  line L261 (478.5317, 87.686) -> (478.4523, 87.7877)
  line L262 (478.4523, 87.7877) -> (478.3801, 87.8947)
  line L263 (478.3801, 87.8947) -> (478.3156, 88.0065)
  line L264 (478.3156, 88.0065) -> (478.259, 88.1225)
  line L265 (478.259, 88.1225) -> (478.2106, 88.2422)
  line L266 (478.2106, 88.2422) -> (478.1708, 88.3649)
  line L267 (478.1708, 88.3649) -> (478.1395, 88.4901)
  line L268 (478.1395, 88.4901) -> (478.1171, 88.6173)
  line L269 (478.1171, 88.6173) -> (478.1036, 88.7456)
  line L270 (478.1036, 88.7456) -> (478.0991, 88.8746)
  line L271 (478.0991, 88.8746) -> (478.1036, 89.0036)
  line L272 (478.1036, 89.0036) -> (478.1171, 89.1319)
  line L273 (478.1171, 89.1319) -> (478.1395, 89.2591)
  line L274 (478.1395, 89.2591) -> (478.1708, 89.3843)
  line L275 (478.1708, 89.3843) -> (478.2106, 89.507)
  line L276 (478.2106, 89.507) -> (478.259, 89.6267)
  line L277 (478.259, 89.6267) -> (478.3156, 89.7427)
  line L278 (478.3156, 89.7427) -> (478.3801, 89.8545)
  line L279 (478.3801, 89.8545) -> (478.4523, 89.9615)
  line L280 (478.4523, 89.9615) -> (478.5317, 90.0632)
  line L281 (478.5317, 90.0632) -> (478.6181, 90.1591)
  line L282 (478.6181, 90.1591) -> (478.7109, 90.2488)
  line L283 (478.7109, 90.2488) -> (478.8098, 90.3317)
  line L284 (478.8098, 90.3317) -> (478.9142, 90.4076)
  line L285 (478.9142, 90.4076) -> (479.0237, 90.476)
  line L286 (479.0237, 90.476) -> (479.1376, 90.5366)
  line L287 (479.1376, 90.5366) -> (479.2555, 90.5891)
  line L288 (479.2555, 90.5891) -> (479.3768, 90.6332)
  line L289 (479.3768, 90.6332) -> (479.5009, 90.6688)
  line L290 (479.5009, 90.6688) -> (479.6271, 90.6956)
  line L291 (479.6271, 90.6956) -> (479.755, 90.7136)
  line L292 (479.755, 90.7136) -> (479.8837, 90.7226)
  line L293 (479.8837, 90.7226) -> (480.0128, 90.7226)
  line L294 (480.0128, 90.7226) -> (480.1415, 90.7136)
  line L295 (480.1415, 90.7136) -> (480.2693, 90.6956)
  line L296 (480.2693, 90.6956) -> (480.3956, 90.6688)
  line L297 (480.3956, 90.6688) -> (480.5196, 90.6332)
  line L298 (480.5196, 90.6332) -> (480.6409, 90.5891)
  line L299 (480.6409, 90.5891) -> (480.7588, 90.5366)
  line L300 (480.7588, 90.5366) -> (480.8728, 90.476)
  line L301 (480.8728, 90.476) -> (480.9823, 90.4076)
  line L302 (480.9823, 90.4076) -> (481.0867, 90.3317)
  line L303 (481.0867, 90.3317) -> (481.1855, 90.2488)
  line L304 (481.1855, 90.2488) -> (481.2784, 90.1591)
  line L305 (481.2784, 90.1591) -> (481.3647, 90.0632)
  line L306 (481.3647, 90.0632) -> (481.4442, 89.9615)
  line L307 (481.4442, 89.9615) -> (481.5164, 89.8545)
  line L308 (481.5164, 89.8545) -> (481.5809, 89.7427)
  line L309 (481.5809, 89.7427) -> (481.6375, 89.6267)
  line L310 (481.6375, 89.6267) -> (481.6858, 89.507)
  line L311 (481.6858, 89.507) -> (481.7257, 89.3843)
  line L312 (481.7257, 89.3843) -> (481.757, 89.2591)
  line L313 (481.757, 89.2591) -> (481.7794, 89.1319)
  line L314 (481.7794, 89.1319) -> (481.7929, 89.0036)
  line L315 (481.7929, 89.0036) -> (481.7974, 88.8746)
  line L316 (577.0956, 89.0397) -> (577.0911, 88.9107)
  line L317 (577.0911, 88.9107) -> (577.0776, 88.7824)
  line L318 (577.0776, 88.7824) -> (577.0552, 88.6552)
  line L319 (577.0552, 88.6552) -> (577.024, 88.53)
  line L320 (577.024, 88.53) -> (576.9841, 88.4073)
  line L321 (576.9841, 88.4073) -> (576.9358, 88.2876)
  line L322 (576.9358, 88.2876) -> (576.8792, 88.1716)
  line L323 (576.8792, 88.1716) -> (576.8146, 88.0598)
  line L324 (576.8146, 88.0598) -> (576.7425, 87.9528)
  line L325 (576.7425, 87.9528) -> (576.663, 87.8511)
  line L326 (576.663, 87.8511) -> (576.5766, 87.7552)
  line L327 (576.5766, 87.7552) -> (576.4838, 87.6655)
  line L328 (576.4838, 87.6655) -> (576.3849, 87.5826)
  line L329 (576.3849, 87.5826) -> (576.2805, 87.5067)
  line L330 (576.2805, 87.5067) -> (576.1711, 87.4383)
  line L331 (576.1711, 87.4383) -> (576.0571, 87.3777)
  line L332 (576.0571, 87.3777) -> (575.9392, 87.3252)
  line L333 (575.9392, 87.3252) -> (575.8179, 87.2811)
  line L334 (575.8179, 87.2811) -> (575.6938, 87.2455)
  line L335 (575.6938, 87.2455) -> (575.5676, 87.2187)
  line L336 (575.5676, 87.2187) -> (575.4398, 87.2007)
  line L337 (575.4398, 87.2007) -> (575.311, 87.1917)
  line L338 (575.311, 87.1917) -> (575.182, 87.1917)
  line L339 (575.182, 87.1917) -> (575.0532, 87.2007)
  line L340 (575.0532, 87.2007) -> (574.9254, 87.2187)
  line L341 (574.9254, 87.2187) -> (574.7992, 87.2455)
  line L342 (574.7992, 87.2455) -> (574.6751, 87.2811)
  line L343 (574.6751, 87.2811) -> (574.5538, 87.3252)
  line L344 (574.5538, 87.3252) -> (574.4359, 87.3777)
  line L345 (574.4359, 87.3777) -> (574.3219, 87.4383)
  line L346 (574.3219, 87.4383) -> (574.2125, 87.5067)
  line L347 (574.2125, 87.5067) -> (574.1081, 87.5826)
  line L348 (574.1081, 87.5826) -> (574.0092, 87.6655)
  line L349 (574.0092, 87.6655) -> (573.9164, 87.7552)
  line L350 (573.9164, 87.7552) -> (573.83, 87.8511)
  line L351 (573.83, 87.8511) -> (573.7505, 87.9528)
  line L352 (573.7505, 87.9528) -> (573.6784, 88.0598)
  line L353 (573.6784, 88.0598) -> (573.6138, 88.1716)
  line L354 (573.6138, 88.1716) -> (573.5572, 88.2876)
  line L355 (573.5572, 88.2876) -> (573.5089, 88.4073)
  line L356 (573.5089, 88.4073) -> (573.469, 88.53)
  line L357 (573.469, 88.53) -> (573.4378, 88.6552)
  line L358 (573.4378, 88.6552) -> (573.4154, 88.7824)
  line L359 (573.4154, 88.7824) -> (573.4019, 88.9107)
  line L360 (573.4019, 88.9107) -> (573.3974, 89.0397)
  line L361 (573.3974, 89.0397) -> (573.4019, 89.1687)
  line L362 (573.4019, 89.1687) -> (573.4154, 89.297)
  line L363 (573.4154, 89.297) -> (573.4378, 89.4242)
  line L364 (573.4378, 89.4242) -> (573.469, 89.5494)
  line L365 (573.469, 89.5494) -> (573.5089, 89.6721)
  line L366 (573.5089, 89.6721) -> (573.5572, 89.7918)
  line L367 (573.5572, 89.7918) -> (573.6138, 89.9078)
  line L368 (573.6138, 89.9078) -> (573.6784, 90.0196)
  line L369 (573.6784, 90.0196) -> (573.7505, 90.1266)
  line L370 (573.7505, 90.1266) -> (573.83, 90.2283)
  line L371 (573.83, 90.2283) -> (573.9164, 90.3242)
  line L372 (573.9164, 90.3242) -> (574.0092, 90.4139)
  line L373 (574.0092, 90.4139) -> (574.1081, 90.4968)
  line L374 (574.1081, 90.4968) -> (574.2125, 90.5727)
  line L375 (574.2125, 90.5727) -> (574.3219, 90.6411)
  line L376 (574.3219, 90.6411) -> (574.4359, 90.7017)
  line L377 (574.4359, 90.7017) -> (574.5538, 90.7542)
  line L378 (574.5538, 90.7542) -> (574.6751, 90.7983)
  line L379 (574.6751, 90.7983) -> (574.7992, 90.8339)
  line L380 (574.7992, 90.8339) -> (574.9254, 90.8607)
  line L381 (574.9254, 90.8607) -> (575.0532, 90.8787)
  line L382 (575.0532, 90.8787) -> (575.182, 90.8877)
  line L383 (575.182, 90.8877) -> (575.311, 90.8877)
  line L384 (575.311, 90.8877) -> (575.4398, 90.8787)
  line L385 (575.4398, 90.8787) -> (575.5676, 90.8607)
  line L386 (575.5676, 90.8607) -> (575.6938, 90.8339)
  line L387 (575.6938, 90.8339) -> (575.8179, 90.7983)
  line L388 (575.8179, 90.7983) -> (575.9392, 90.7542)
  line L389 (575.9392, 90.7542) -> (576.0571, 90.7017)
  line L390 (576.0571, 90.7017) -> (576.1711, 90.6411)
  line L391 (576.1711, 90.6411) -> (576.2805, 90.5727)
  line L392 (576.2805, 90.5727) -> (576.3849, 90.4968)
  line L393 (576.3849, 90.4968) -> (576.4838, 90.4139)
  line L394 (576.4838, 90.4139) -> (576.5766, 90.3242)
  line L395 (576.5766, 90.3242) -> (576.663, 90.2283)
  line L396 (576.663, 90.2283) -> (576.7425, 90.1266)
  line L397 (576.7425, 90.1266) -> (576.8146, 90.0196)
  line L398 (576.8146, 90.0196) -> (576.8792, 89.9078)
  line L399 (576.8792, 89.9078) -> (576.9358, 89.7918)
  line L400 (576.9358, 89.7918) -> (576.9841, 89.6721)
  line L401 (576.9841, 89.6721) -> (577.024, 89.5494)
  line L402 (577.024, 89.5494) -> (577.0552, 89.4242)
  line L403 (577.0552, 89.4242) -> (577.0776, 89.297)
  line L404 (577.0776, 89.297) -> (577.0911, 89.1687)
  line L405 (577.0911, 89.1687) -> (577.0956, 89.0397)
  line L406 (577.0956, 18.1204) -> (577.0911, 17.9914)
  line L407 (577.0911, 17.9914) -> (577.0776, 17.863)
  line L408 (577.0776, 17.863) -> (577.0552, 17.7359)
  line L409 (577.0552, 17.7359) -> (577.024, 17.6107)
  line L410 (577.024, 17.6107) -> (576.9841, 17.4879)
  line L411 (576.9841, 17.4879) -> (576.9358, 17.3683)
  line L412 (576.9358, 17.3683) -> (576.8792, 17.2523)
  line L413 (576.8792, 17.2523) -> (576.8146, 17.1405)
  line L414 (576.8146, 17.1405) -> (576.7425, 17.0335)
  line L415 (576.7425, 17.0335) -> (576.663, 16.9318)
  line L416 (576.663, 16.9318) -> (576.5766, 16.8359)
  line L417 (576.5766, 16.8359) -> (576.4838, 16.7462)
  line L418 (576.4838, 16.7462) -> (576.3849, 16.6632)
  line L419 (576.3849, 16.6632) -> (576.2805, 16.5874)